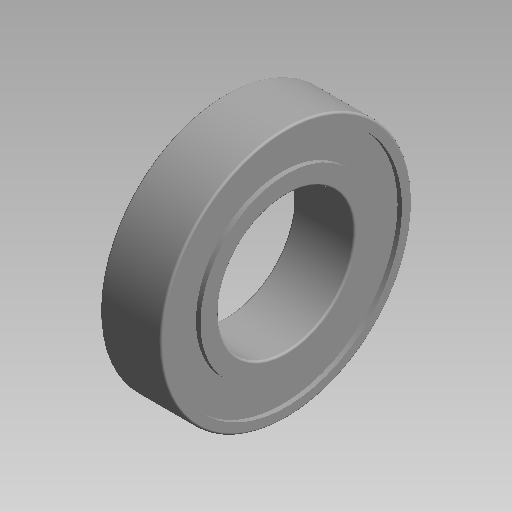
# Autodesk Inventor part: bearing_6904
Saved by Autodesk Inventor 2021.2 (Build 252289000, 289)
## iProperties
Part Number: bearing_6904
Material: 一般
Catalog Web Link: www.cadenas.de
Description: 6000_bearing-Deep Groove Ball Bearings
Vendor: MISUMI
Document SubType Name: Modeling
Designer: partserver
Manufacturer: MISUMI
Mass: 6.32096 g
Surface Area: 33.3022 cm^2
Volume: 6.32096 cm^3
Density: 1 g/cm^3
Appearance: PSOLRGB-192-192-192
Category: PARTsolutions
Company: MISUMI
PSOL_IDENT_0: {$CADENAS_DATA\23d-libs\misumi\metric\accessories\bearing_6000.prj},171 {VTYP=3D},{NB=bearing_6904},
PSOL_IDENT_1: {LINA=bearing_6904},{NN=6000_bearing},{DATE=30.06.2021 13:30:08},{GEOMDATE=24.10.2013 00:00:00},{VER
PSOL_IDENT_2: SION=},{LINEID=220},{WBVAR=},{WBNUMERIC=}  {NB=bearing_6904},{LINA=bearing_6904},{KT=DUMMY},{PN=bear
PSOL_IDENT_3: ing_6904},{BN=6904},{DD=20},{D=37},{B=9},{RR=0.3},{DSMIN=22.0},{DS1=24.00},{DSMAX=24.00},{DDHH=35.0}
PSOL_IDENT_4: ,{R=0.3},{R1=0.250},{R2=0.300},{MASS=36},{MASS11=36},{AA=7.7000},{BB=1.5000},{CC=2.7000},{DD1=35.700
PSOL_IDENT_5: }
NB: bearing_6904
NN: 6000_bearing
NT: Deep Groove Ball Bearings
NBSYN: $PN.
LINA: bearing_6904
CATALOG: Misumi
PN: bearing_6904
BN: 6904
DD: 20
D: 37
B: 9
RR: 0.3
DSMIN: 22
DDHH: 35
R: 0.3
MASS11: 36
SUPPLIER: MISUMI
ARTICLENO: bearing_6904
BOMINFO: bearing_6904
CREATOR: CADENAS GmbH
d1: 0.000 mm
Title: bearing_6904
Author: Cadenas PARTsolutions
Comments: Deep Groove Ball Bearings
Autodesk Inventor part; units mm, degrees
sketch "Sketch_1" plane through (0, 0, 0) normal (0, 0, 1) x (1, 0, 0)
  line L0 (9, 0) -> (0, 0)
  arc A0 (0, 10.3) -> (0.3, 10) centre (0.3, 10.3) ccw
  line L1 (0.3, 10) -> (8.7, 10)
  arc A1 (8.7, 10) -> (9, 10.3) centre (8.7, 10.3) ccw
  line L2 (9, 10.3) -> (9, 12.7)
  line L3 (9, 12.7) -> (8.35, 12.7)
  line L4 (8.35, 12.7) -> (8.35, 17)
  line L5 (8.35, 17) -> (9, 17)
  line L6 (9, 17) -> (9, 18.2)
  arc A2 (9, 18.2) -> (8.7, 18.5) centre (8.7, 18.2) ccw
  line L7 (8.7, 18.5) -> (0.3, 18.5)
  arc A3 (0.3, 18.5) -> (0, 18.2) centre (0.3, 18.2) ccw
  line L8 (0, 18.2) -> (0, 17)
  line L9 (0, 17) -> (0.65, 17)
  line L10 (0.65, 17) -> (0.65, 12.7)
  line L11 (0.65, 12.7) -> (0, 12.7)
  line L12 (0, 12.7) -> (0, 10.3)
  constraints: 26 end point, 8 point on circle, 4 centre point
revolve "Revolution1" add sketch "Sketch_1" angle 360 about axis through (9, 0, 0) along (1, 0, 0)
ref_plane "center_point_XY" through (4.5, 0, 0) normal (1, 0, 0) x (0, 0, -1)
ref_plane "center_point_YZ" through (4.5, 0, 0) normal (0, 0, -1) x (0, 1, 0)
ref_plane "center_point_ZX" through (4.5, 0, 0) normal (0, 1, 0) x (1, 0, 0)
ref_plane "to_housing_XY" through (0, 0, 0) normal (1, 0, 0) x (0, 0, -1)
ref_plane "to_housing_YZ" through (0, 0, 0) normal (0, 0, -1) x (0, 1, 0)
ref_plane "to_housing_ZX" through (0, 0, 0) normal (0, 1, 0) x (1, 0, 0)
ref_plane "to_ring_XY" through (7.7, 0, 0) normal (1, 0, 0) x (0, 0, -1)
ref_plane "to_ring_YZ" through (7.7, 0, 0) normal (0, 0, -1) x (0, 1, 0)
ref_plane "to_ring_ZX" through (7.7, 0, 0) normal (0, 1, 0) x (1, 0, 0)
body "Solid1"
